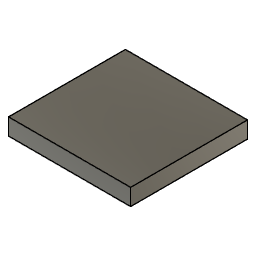
cam v1 (Autodesk Fusion 360 design; units mm, degrees)
Autodesk Fusion 360 part; units mm, degrees
note: some values were not read from the file. Set by a fixed rule: which face or edge a step refers to.
sketch "Sketch1" plane through (0, 0, 0) normal (0, 0, 1) x (1, 0, 0)
  line L0 (0, 0) -> (37.9, 0)
  line L1 (37.9, 0) -> (37.9, 38.1)
  line L2 (37.9, 38.1) -> (0, 38.1)
  line L3 (0, 38.1) -> (0, 0)
  line L4 (-2, 40.1) -> (39.9, 40.1)
  line L5 (39.9, 40.1) -> (39.9, -2)
  line L6 (39.9, -2) -> (-2, -2)
  line L7 (-2, -2) -> (-2, 40.1)
  dimension "d3" = 2
  dimension "d5" = 2
  dimension "d6" = 2
  dimension "d7" = 2
  constraint horizontal L0
  constraint vertical L1
  constraint horizontal L2
  constraint vertical L3
  constraint coincident L0.start L3.end
  constraint horizontal L4
  constraint vertical L5
  constraint horizontal L6
  constraint vertical L7
  measures "d3" distance of L1 L5
  measures "d5" distance of L3 L7
  measures "d6" distance of L2 L4
  measures "d7" distance of L0 L6
sketch "Sketch2" plane through (0, 40.1, 0) normal (0, 1, 0) x (-1, 0, 0)
sketch "Sketch3" plane through (0, 0, 0) normal (1, 0, 0) x (0, 1, 0)
  line L0 (38.1, -0.1) -> (38.1, 0)
  line L1 (0, 0) -> (0, -0.1)
  line L2 (0, -0.1) -> (38.1, -0.1)
  line L3 (38.1, 0.383) -> (0, 0.383)
  line L4 (0, 0.383) -> (0, 1.1)
  line L5 (0, 1.1) -> (38.1, 1.1)
  line L6 (38.1, 1.1) -> (38.1, 0.383)
  line L7 (38.1, 0) -> (0, 0)
  constraint horizontal L3
  constraint vertical L4
  constraint horizontal L5
  constraint vertical L6
  constraint coincident L0 L3.start
ref_plane "WorkPlane1" through (18.95, 19.05, -0.05) normal (-1, 0, 0) x (0, 1, 0)
sketch "Sketch4" plane through (0, 0, 0) normal (1, 0, 0) x (0, 1, 0)
sketch "Sketch5" plane through (0, 0, 0) normal (0, 0, 1) x (1, 0, 0)
  line L0 (0, 0) -> (37.9, 0)
  line L1 (37.9, 0) -> (37.9, -38.1)
  line L2 (37.9, -38.1) -> (0, -38.1)
  line L3 (0, -38.1) -> (0, 0)
  dimension "d19" = 37.9
  dimension "d20" = 38.1
  constraint horizontal L0
  constraint vertical L1
  constraint horizontal L2
  constraint vertical L3
  constraint coincident L0.start L3.end
  measures "d19" distance of L0.start L0.end
  measures "d20" distance of L0.start L2.end
extrude "Extrude5" add sketch "Sketch5" along normal blind 2 makes body 1
extrude "Extrude6" add 1 faces at (37.9, -12.7, 0.6667) along direction (1, 0, 0) blind 2 separate body on bodies 1 makes body 2
extrude "Extrude7" add 1 faces at (0, -25.4, 0.6667) along direction (-1, 0, 0) blind 2 separate body on bodies 1 makes body 3
extrude "Extrude8" add 3 faces at (38.5667, -38.1, 0.6667) (25.2667, -38.1, 0.6667) (-0.6667, -38.1, 0.6667) along direction (0, -1, 0) blind 2 separate body on bodies 1 2 3 makes body 4
extrude "Extrude9" add 5 faces at (-0.6667, -25.4, 0) (38.5667, -38.7667, 0) (-0.6667, -38.7667, 0) (25.2667, -38.7667, 0) (38.5667, -12.7, 0) along direction (0, 0, -1) blind 2.7 on bodies 2 3 4 bodies 3 2 1 4
sketch "Sketch6" plane through (0, 0, -2.7) normal (0, 0, -1) x (1, 0, 0)
  line L0 (0, 0) -> (0, 38.1)
  line L1 (0, 38.1) -> (37.9, 38.1)
  line L2 (37.9, 38.1) -> (37.9, 0)
  line L3 (37.9, 0) -> (39.9, 0)
  line L4 (39.9, 0) -> (39.9, 40.1)
  line L5 (39.9, 40.1) -> (-2, 40.1)
  line L6 (-2, 40.1) -> (-2, 0)
  line L7 (-2, 0) -> (0, 0)
  line L8 (-2, 40.1) -> (8, 40.1)
  line L9 (8, 0) -> (-2, 0)
  line L10 (-2, 0) -> (-2, 40.1)
  line L11 (39.9, 0) -> (29.9, 0)
  line L12 (29.9, 40.1) -> (39.9, 40.1)
  line L13 (39.9, 40.1) -> (39.9, 0)
  line L14 (-2, 40.1) -> (39.9, 40.1)
  line L15 (39.9, 40.1) -> (39.9, 30.1)
  line L16 (-2, 30.1) -> (-2, 40.1)
  line L17 (8, 30.1) -> (8, 0)
  line L18 (29.9, 30.1) -> (8, 30.1)
  line L19 (29.9, 0) -> (29.9, 30.1)
  dimension "d31" = 10
  dimension "d32" = 10
  constraint horizontal L8
  constraint horizontal L9
  constraint vertical L10
  constraint coincident L5.end L6.start
  constraint horizontal L11
  constraint vertical L19
  constraint horizontal L12
  constraint vertical L13
  constraint coincident L3.end L4.start
  constraint horizontal L14
  constraint vertical L15
  constraint vertical L16
  measures "d31" distance of L3.end L11.end
  measures "d32" distance of L5.end L16.start
extrude "Extrude10" add sketch "Sketch6" along normal blind 1 bodies 3
